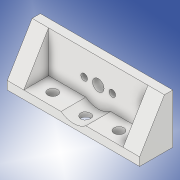
# Autodesk Inventor part: C005
Saved by Autodesk Inventor 2017 (Build 210142000, 142)
## iProperties
Created: 2017-06-13
Part Number: C005
Material: ABS Plastic
Document SubType Name: Modeling
Designer: zallen
Density: 1.06 g/cm^3
Appearance: CR White
Mass: 67.5643 g
Surface Area: 46.2838 cm^2
Volume: 8.60691 cm^3
Author: zallen
Autodesk Inventor part; units mm, degrees
ref_plane "YZ Plane" through (0, 0, 0) normal (1, 0, 0) x (0, 1, 0)
ref_plane "XZ Plane" through (0, 0, 0) normal (0, 1, 0) x (-1, 0, 0)
ref_plane "XY Plane" through (0, 0, 0) normal (0, 0, 1) x (1, 0, 0)
sketch "Sketch1" plane through (0, 0, 0) normal (0, 0, 1) x (1, 0, 0)
  line L0 (0, 0) -> (80, 0)
  circle A0 centre (40, 15) radius 3.5
  line L1 (0, 0) -> (0, 30)
  line L2 (0, 30) -> (80, 30)
  line L3 (80, 30) -> (80, 0)
  point P0 (40, 0)
  dimension "d0" = 80
  dimension "d2" = 7
  dimension "d3" = 15
  dimension "d4" = 30
  constraints: 8 end point, 2 perpendicular, 1 centre point, 1 horizontal, 1 midpoint, 1 vertical, 1 vertical alignment
  measures "d0" distance of L0.start L0.end
  measures "d2" diameter of A0
  measures "d3" distance of point (40, 0) A0.centre
  measures "d4" distance of L0.start L1.end
extrude "Extrusion1" add sketch "Sketch1" along normal blind 5
sketch "Sketch2" plane through (0, 0, 5) normal (0, 0, 1) x (1, 0, 0)
  line L0 (0, 0) -> (80, 0) projected
  line L1 (0, 0) -> (80, 0)
  line L2 (80, 0) -> (80, 5)
  line L3 (80, 5) -> (0, 5)
  line L4 (0, 5) -> (0, 0)
  line L5 (80, 0) -> (80, 30) projected
  point P0 (40, 0)
  dimension "d8" = 5
  constraints: 8 end point, 2 midpoint, 2 parallel, 2 point on line, 1 horizontal, 1 perpendicular
  measures "d8" distance of L1.end L2.end
extrude "Extrusion2" add sketch "Sketch2" along normal blind 15
sketch "Sketch3" plane through (0, 0, 5) normal (0, 0, 1) x (1, 0, 0)
  circle A0 centre (31.5, 15) radius 2
  circle A1 centre (48.5, 15) radius 2
  line L0 (80, 5) -> (80, 30) projected
  line L1 (80, 30) -> (0, 30) projected
  line L2 (0, 30) -> (0, 5) projected
  line L3 (0, 5) -> (80, 5) projected
  circle A2 centre (40, 15) radius 3.5 projected
  line L4 (31.5, 15) -> (48.5, 15) construction
  point P0 (0, 0)
  dimension "d11" = 4
  dimension "d12" = 4
  dimension "d13" = 17
  constraints: 2 centre point, 2 end point, 1 coincident, 1 horizontal, 1 horizontal alignment, 1 midpoint
  measures "d11" diameter of A0
  measures "d12" diameter of A1
  measures "d13" distance of L4.end L4.start
extrude "Extrusion3" cut sketch "Sketch3" against normal through all contours A0 | A1
sketch "Sketch5" plane through (0, 5, 5) normal (0, 1, 0) x (1, 0, 0)
  line L0 (0, 0) -> (0, -15) construction
  line L1 (80, 5) -> (80, -15) construction
  circle A0 centre (20, -7.5) radius 3
  circle A1 centre (40, -7.5) radius 3
  circle A2 centre (60, -7.5) radius 3
  line L2 (0, -7.5) -> (80, -7.5) construction
  point P0 (0, 5)
  point P1 (40, -7.5)
  point P2 (40, -7.5)
  dimension "d17" = 6
  dimension "d18" = 6
  dimension "d19" = 20
  dimension "d25" = 6
  dimension "d26" = 20
  constraints: 3 centre point, 3 point on line, 2 end point, 2 midpoint, 1 coincident, 1 perpendicular
  measures "d17" diameter of A0
  measures "d18" diameter of A1
  measures "d19" distance of A1.centre A0.centre
  measures "d25" diameter of A2
  measures "d26" distance of A2.centre A1.centre
extrude "Extrusion4" cut sketch "Sketch5" against normal through all
sketch "Sketch6" plane through (0, 0, 5) normal (0, 0, 1) x (1, 0, 0)
  circle A0 centre (40, 15) radius 3.5 projected
  circle A1 centre (40, 15) radius 12.5
  point P0 (0, 0)
  dimension "d27" = 25
  constraints: 1 centre point, 1 coincident
  measures "d27" diameter of A1
extrude "Extrusion5" cut sketch "Sketch6" along normal through all
sketch "Sketch8" plane through (80, 0, 0) normal (1, 0, 0) x (0, 0, -1)
  line L0 (-5, 5) -> (-20, 5) projected
  line L1 (-5, 5) -> (-5, 30) projected
  line L2 (-20, 5) -> (-5, 30)
  line L3 (-5, 30) -> (-5, 5)
  line L4 (-5, 5) -> (-20, 5)
  point P0 (0, 0)
  constraints: 6 end point, 1 collinear, 1 perpendicular
extrude "Extrusion6" add sketch "Sketch8" against normal blind 10
sketch "Sketch9" plane through (0, 0, 0) normal (-1, 0, 0) x (0, 0, 1)
  line L0 (20, 0) -> (20, 5) projected
  line L1 (20, 5) -> (5, 30)
  line L2 (5, 5) -> (20, 5) projected
  line L3 (5, 30) -> (5, 5)
  line L4 (5, 5) -> (20, 5)
  point P0 (0, 0)
  constraints: 6 end point, 1 collinear, 1 perpendicular
extrude "Extrusion7" add sketch "Sketch9" against normal blind 10
body "Solid1"
